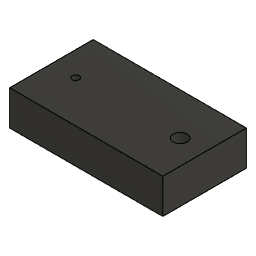
VL53L0X v1 (Autodesk Fusion 360 design; units mm, degrees)
Autodesk Fusion 360 part; units mm, degrees
sketch "Sketch1" plane through (0, 0, 0) normal (0, 0, 1) x (1, 0, 0)
  line L0 (-2.2, 1.2) -> (2.2, 1.2)
  line L1 (2.2, 1.2) -> (2.2, -1.2)
  line L2 (2.2, -1.2) -> (-2.2, -1.2)
  line L3 (-2.2, -1.2) -> (-2.2, 1.2)
  circle A0 centre (-1.5, 0) radius 0.1
  circle A1 centre (1.5, 0) radius 0.2
  dimension "d3" = 0.2
  dimension "d4" = 0.4
  constraint horizontal L0
  constraint vertical L1
  constraint horizontal L2
  constraint vertical L3
  measures "d3" diameter of A0
  measures "d4" diameter of A1
extrude "Extrude1" add sketch "Sketch1" along normal blind 1
